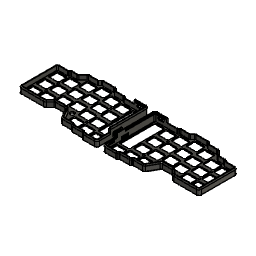
mriya-bumper-mjf-v1.01 (Autodesk Fusion 360 design; units mm, degrees)
Autodesk Fusion 360 part; units mm, degrees
(part 1 of 2)
sketch "mriya" plane through (0, 0, 0) normal (0, 0, 1) x (1, 0, 0)
  line L0 (-101.0213, 15.6719) -> (-94.7787, 21.9145) construction
  line L1 (-26.4858, 1.079) -> (-27.6142, 2.2074) construction
  line L2 (-138.1, 14.7932) -> (-103.1426, 14.7932) construction
  line L3 (-44.0716, 2.7932) -> (-29.0284, 2.7932) construction
  line L4 (-8.6, 0.4932) -> (-25.0716, 0.4932) construction
  line L5 (-64.4741, 6.1094) -> (-72.7517, 20.7608) construction
  line L6 (-45.4858, 3.379) -> (-46.6142, 4.5074) construction
  line L7 (-122.6142, 71.579) -> (-121.4858, 72.7074) construction
  line L8 (-101.0716, 81.2932) -> (-87.2284, 81.2932) construction
  line L9 (-138.1, 70.9932) -> (-124.0284, 70.9932) construction
  line L10 (-92.6574, 22.7932) -> (-76.2344, 22.7932) construction
  line L11 (-48.0284, 5.0932) -> (-62.7328, 5.0932) construction
  line L12 (-82.0716, 84.7932) -> (-64.7284, 84.7932) construction
  line L13 (-58.5716, 80.2932) -> (-45.7284, 80.2932) construction
  line L14 (-24.1, 19.4932) -> (-7.1, 19.4932) construction
  line L15 (-25.6, 20.9932) -> (-25.6, 77.9932) construction
  line L16 (-83.4858, 84.2074) -> (-85.8142, 81.879) construction
  line L17 (-63.3142, 84.2074) -> (-59.9858, 80.879) construction
  line L18 (-139.6, 69.4932) -> (-139.6, 16.2932) construction
  line L19 (-43.1858, 78.579) -> (-44.3142, 79.7074) construction
  line L20 (-99.4, 40.3932) -> (-99.4, 27.9932) construction
  line L21 (-98.6, 41.1932) -> (-86.2, 41.1932) construction
  line L22 (-98.6, 27.1932) -> (-86.2, 27.1932) construction
  line L23 (-85.4, 40.3932) -> (-85.4, 27.9932) construction
  line L24 (-42.4, 56.0932) -> (-42.4, 43.6932) construction
  line L25 (-41.6, 56.8932) -> (-29.2, 56.8932) construction
  line L26 (-41.6, 42.8932) -> (-29.2, 42.8932) construction
  line L27 (-28.4, 56.0932) -> (-28.4, 43.6932) construction
  line L28 (-61.4, 58.3932) -> (-61.4, 45.9932) construction
  line L29 (-60.6, 59.1932) -> (-48.2, 59.1932) construction
  line L30 (-60.6, 45.1932) -> (-48.2, 45.1932) construction
  line L31 (-47.4, 58.3932) -> (-47.4, 45.9932) construction
  line L32 (-137.4, 68.0932) -> (-137.4, 55.6932) construction
  line L33 (-136.6, 68.8932) -> (-124.2, 68.8932) construction
  line L34 (-136.6, 54.8932) -> (-124.2, 54.8932) construction
  line L35 (-123.4, 68.0932) -> (-123.4, 55.6932) construction
  line L36 (-61.4, 39.3932) -> (-61.4, 26.9932) construction
  line L37 (-60.6, 40.1932) -> (-48.2, 40.1932) construction
  line L38 (-60.6, 26.1932) -> (-48.2, 26.1932) construction
  line L39 (-47.4, 39.3932) -> (-47.4, 26.9932) construction
  line L40 (-42.4, 18.0932) -> (-42.4, 5.6932) construction
  line L41 (-41.6, 18.8932) -> (-29.2, 18.8932) construction
  line L42 (-41.6, 4.8932) -> (-29.2, 4.8932) construction
  line L43 (-28.4, 18.0932) -> (-28.4, 5.6932) construction
  line L44 (-23.4, 15.7932) -> (-23.4, 3.3932) construction
  line L45 (-22.6, 16.5932) -> (-10.2, 16.5932) construction
  line L46 (-22.6, 2.5932) -> (-10.2, 2.5932) construction
  line L47 (-9.4, 15.7932) -> (-9.4, 3.3932) construction
  line L48 (-137.4, 49.0932) -> (-137.4, 36.6932) construction
  line L49 (-136.6, 49.8932) -> (-124.2, 49.8932) construction
  line L50 (-136.6, 35.8932) -> (-124.2, 35.8932) construction
  line L51 (-123.4, 49.0932) -> (-123.4, 36.6932) construction
  line L52 (-118.4, 51.3932) -> (-118.4, 38.9932) construction
  line L53 (-117.6, 52.1932) -> (-105.2, 52.1932) construction
  line L54 (-117.6, 38.1932) -> (-105.2, 38.1932) construction
  line L55 (-104.4, 51.3932) -> (-104.4, 38.9932) construction
  line L56 (-137.4, 30.0932) -> (-137.4, 17.6932) construction
  line L57 (-136.6, 30.8932) -> (-124.2, 30.8932) construction
  line L58 (-136.6, 16.8932) -> (-124.2, 16.8932) construction
  line L59 (-123.4, 30.0932) -> (-123.4, 17.6932) construction
  line L60 (-61.4, 20.3932) -> (-61.4, 7.9932) construction
  line L61 (-60.6, 21.1932) -> (-48.2, 21.1932) construction
  line L62 (-60.6, 7.1932) -> (-48.2, 7.1932) construction
  line L63 (-47.4, 20.3932) -> (-47.4, 7.9932) construction
  line L64 (-80.4, 43.8932) -> (-80.4, 31.4932) construction
  line L65 (-79.6, 44.6932) -> (-67.2, 44.6932) construction
  line L66 (-79.6, 30.6932) -> (-67.2, 30.6932) construction
  line L67 (-66.4, 43.8932) -> (-66.4, 31.4932) construction
  line L68 (-80.4, 81.8932) -> (-80.4, 69.4932) construction
  line L69 (-79.6, 82.6932) -> (-67.2, 82.6932) construction
  line L70 (-79.6, 68.6932) -> (-67.2, 68.6932) construction
  line L71 (-66.4, 81.8932) -> (-66.4, 69.4932) construction
  line L72 (-42.4, 37.0932) -> (-42.4, 24.6932) construction
  line L73 (-41.6, 37.8932) -> (-29.2, 37.8932) construction
  line L74 (-41.6, 23.8932) -> (-29.2, 23.8932) construction
  line L75 (-28.4, 37.0932) -> (-28.4, 24.6932) construction
  line L76 (-118.4, 32.3932) -> (-118.4, 19.9932) construction
  line L77 (-117.6, 33.1932) -> (-105.2, 33.1932) construction
  line L78 (-117.6, 19.1932) -> (-105.2, 19.1932) construction
  line L79 (-104.4, 32.3932) -> (-104.4, 19.9932) construction
  line L80 (-61.4, 77.3932) -> (-61.4, 64.9932) construction
  line L81 (-60.6, 78.1932) -> (-48.2, 78.1932) construction
  line L82 (-60.6, 64.1932) -> (-48.2, 64.1932) construction
  line L83 (-47.4, 77.3932) -> (-47.4, 64.9932) construction
  line L84 (-42.4, 75.0932) -> (-42.4, 62.6932) construction
  line L85 (-41.6, 75.8932) -> (-29.2, 75.8932) construction
  line L86 (-41.6, 61.8932) -> (-29.2, 61.8932) construction
  line L87 (-28.4, 75.0932) -> (-28.4, 62.6932) construction
  line L88 (-118.4, 70.3932) -> (-118.4, 57.9932) construction
  line L89 (-117.6, 71.1932) -> (-105.2, 71.1932) construction
  line L90 (-117.6, 57.1932) -> (-105.2, 57.1932) construction
  line L91 (-104.4, 70.3932) -> (-104.4, 57.9932) construction
  line L92 (-99.4, 59.3932) -> (-99.4, 46.9932) construction
  line L93 (-98.6, 60.1932) -> (-86.2, 60.1932) construction
  line L94 (-98.6, 46.1932) -> (-86.2, 46.1932) construction
  line L95 (-85.4, 59.3932) -> (-85.4, 46.9932) construction
  line L96 (-80.4, 62.8932) -> (-80.4, 50.4932) construction
  line L97 (-79.6, 63.6932) -> (-67.2, 63.6932) construction
  line L98 (-79.6, 49.6932) -> (-67.2, 49.6932) construction
  line L99 (-66.4, 62.8932) -> (-66.4, 50.4932) construction
  line L100 (-99.4, 78.3932) -> (-99.4, 65.9932) construction
  line L101 (-98.6, 79.1932) -> (-86.2, 79.1932) construction
  line L102 (-98.6, 65.1932) -> (-86.2, 65.1932) construction
  line L103 (-85.4, 78.3932) -> (-85.4, 65.9932) construction
  circle A0 centre (-120.9, 53.5432) radius 1.6
  circle A1 centre (-120.9, 34.5432) radius 1.6
  circle A2 centre (-68.5, 23.5932) radius 3.5
  circle A3 centre (-44.9, 22.5432) radius 1.6
  circle A4 centre (-44.9, 60.5432) radius 1.6
  arc A5 (-43.1858, 78.579) -> (-41.7716, 77.9932) centre (-41.7716, 79.9932) ccw construction
  arc A6 (-44.3142, 79.7074) -> (-45.7284, 80.2932) centre (-45.7285, 78.2931) ccw construction
  arc A7 (-59.9858, 80.879) -> (-58.5716, 80.2932) centre (-58.5716, 82.2931) ccw construction
  arc A8 (-63.3142, 84.2074) -> (-64.7284, 84.7932) centre (-64.7285, 82.7931) ccw construction
  arc A9 (-82.0716, 84.7932) -> (-83.4858, 84.2074) centre (-82.0716, 82.7933) ccw construction
  arc A10 (-87.2284, 81.2932) -> (-85.8142, 81.879) centre (-87.2284, 83.2932) ccw construction
  arc A11 (-101.0716, 81.2932) -> (-102.4858, 80.7074) centre (-101.0716, 79.2933) ccw construction
  arc A12 (-120.0716, 73.2932) -> (-121.4858, 72.7074) centre (-120.0716, 71.2933) ccw construction
  arc A13 (-124.0284, 70.9932) -> (-122.6142, 71.579) centre (-124.0284, 72.9932) ccw construction
  arc A14 (-138.1, 70.9932) -> (-139.6, 69.4932) centre (-138.1, 69.4932) ccw construction
  arc A15 (-139.6, 16.2932) -> (-138.1, 14.7932) centre (-138.1, 16.2932) ccw construction
  arc A16 (-103.1426, 14.7932) -> (-101.0213, 15.6719) centre (-103.1426, 17.7931) ccw construction
  arc A17 (-92.6574, 22.7932) -> (-94.7787, 21.9145) centre (-92.6573, 19.7931) ccw construction
  arc A18 (-72.7517, 20.7608) -> (-76.2344, 22.7932) centre (-76.2344, 18.793) ccw construction
  arc A19 (-64.4741, 6.1094) -> (-62.7328, 5.0932) centre (-62.7328, 7.0932) ccw construction
  arc A20 (-46.6142, 4.5074) -> (-48.0284, 5.0932) centre (-48.0284, 3.0933) ccw construction
  arc A21 (-45.4858, 3.379) -> (-44.0716, 2.7932) centre (-44.0715, 4.7933) ccw construction
  arc A22 (-27.6142, 2.2074) -> (-29.0284, 2.7932) centre (-29.0284, 0.7933) ccw construction
  arc A23 (-26.4858, 1.079) -> (-25.0716, 0.4932) centre (-25.0715, 2.4933) ccw construction
  arc A24 (-8.6, 0.4932) -> (-7.1, 1.9932) centre (-8.6, 1.9932) ccw construction
  arc A25 (-25.6, 20.9932) -> (-24.1, 19.4932) centre (-24.1, 20.9932) ccw construction
  line L104 (-7.1, 1.9932) -> (-7.1, 76.4932) construction
  line L105 (-41.7716, 77.9932) -> (-8.6, 77.9932) construction
  arc A26 (-7.1, 76.4932) -> (-8.6, 77.9932) centre (-8.6, 76.4932) ccw construction
  arc A27 (-136.6, 68.8932) -> (-137.4, 68.0932) centre (-136.6, 68.0932) ccw construction
  arc A28 (-123.4, 68.0932) -> (-124.2, 68.8932) centre (-124.2, 68.0932) ccw construction
  arc A29 (-124.2, 54.8932) -> (-123.4, 55.6932) centre (-124.2, 55.6932) ccw construction
  arc A30 (-137.4, 55.6932) -> (-136.6, 54.8932) centre (-136.6, 55.6932) ccw construction
  arc A31 (-136.6, 49.8932) -> (-137.4, 49.0932) centre (-136.6, 49.0932) ccw construction
  arc A32 (-123.4, 49.0932) -> (-124.2, 49.8932) centre (-124.2, 49.0932) ccw construction
  arc A33 (-124.2, 35.8932) -> (-123.4, 36.6932) centre (-124.2, 36.6932) ccw construction
  arc A34 (-137.4, 36.6932) -> (-136.6, 35.8932) centre (-136.6, 36.6932) ccw construction
  arc A35 (-136.6, 30.8932) -> (-137.4, 30.0932) centre (-136.6, 30.0932) ccw construction
  arc A36 (-123.4, 30.0932) -> (-124.2, 30.8932) centre (-124.2, 30.0932) ccw construction
  arc A37 (-124.2, 16.8932) -> (-123.4, 17.6932) centre (-124.2, 17.6932) ccw construction
  arc A38 (-137.4, 17.6932) -> (-136.6, 16.8932) centre (-136.6, 17.6932) ccw construction
  arc A39 (-118.4, 19.9932) -> (-117.6, 19.1932) centre (-117.6, 19.9932) ccw construction
  arc A40 (-105.2, 19.1932) -> (-104.4, 19.9932) centre (-105.2, 19.9932) ccw construction
  arc A41 (-104.4, 32.3932) -> (-105.2, 33.1932) centre (-105.2, 32.3932) ccw construction
  arc A42 (-117.6, 33.1932) -> (-118.4, 32.3932) centre (-117.6, 32.3932) ccw construction
  arc A43 (-105.2, 38.1932) -> (-104.4, 38.9932) centre (-105.2, 38.9932) ccw construction
  arc A44 (-118.4, 38.9932) -> (-117.6, 38.1932) centre (-117.6, 38.9932) ccw construction
  arc A45 (-117.6, 52.1932) -> (-118.4, 51.3932) centre (-117.6, 51.3932) ccw construction
  arc A46 (-104.4, 51.3932) -> (-105.2, 52.1932) centre (-105.2, 51.3932) ccw construction
  arc A47 (-118.4, 57.9932) -> (-117.6, 57.1932) centre (-117.6, 57.9932) ccw construction
  arc A48 (-105.2, 57.1932) -> (-104.4, 57.9932) centre (-105.2, 57.9932) ccw construction
  arc A49 (-104.4, 70.3932) -> (-105.2, 71.1932) centre (-105.2, 70.3932) ccw construction
  arc A50 (-117.6, 71.1932) -> (-118.4, 70.3932) centre (-117.6, 70.3932) ccw construction
  arc A51 (-98.6, 79.1932) -> (-99.4, 78.3932) centre (-98.6, 78.3932) ccw construction
  arc A52 (-85.4, 78.3932) -> (-86.2, 79.1932) centre (-86.2, 78.3932) ccw construction
  arc A53 (-86.2, 65.1932) -> (-85.4, 65.9932) centre (-86.2, 65.9932) ccw construction
  arc A54 (-99.4, 65.9932) -> (-98.6, 65.1932) centre (-98.6, 65.9932) ccw construction
  arc A55 (-98.6, 60.1932) -> (-99.4, 59.3932) centre (-98.6, 59.3932) ccw construction
  arc A56 (-85.4, 59.3932) -> (-86.2, 60.1932) centre (-86.2, 59.3932) ccw construction
  arc A57 (-86.2, 46.1932) -> (-85.4, 46.9932) centre (-86.2, 46.9932) ccw construction
  arc A58 (-99.4, 46.9932) -> (-98.6, 46.1932) centre (-98.6, 46.9932) ccw construction
  arc A59 (-98.6, 41.1932) -> (-99.4, 40.3932) centre (-98.6, 40.3932) ccw construction
  arc A60 (-99.4, 27.9932) -> (-98.6, 27.1932) centre (-98.6, 27.9932) ccw construction
  arc A61 (-86.2, 27.1932) -> (-85.4, 27.9932) centre (-86.2, 27.9932) ccw construction
  arc A62 (-85.4, 40.3932) -> (-86.2, 41.1932) centre (-86.2, 40.3932) ccw construction
  arc A63 (-80.4, 31.4932) -> (-79.6, 30.6932) centre (-79.6, 31.4932) ccw construction
  arc A64 (-79.6, 44.6932) -> (-80.4, 43.8932) centre (-79.6, 43.8932) ccw construction
  arc A65 (-66.4, 43.8932) -> (-67.2, 44.6932) centre (-67.2, 43.8932) ccw construction
  arc A66 (-67.2, 30.6932) -> (-66.4, 31.4932) centre (-67.2, 31.4932) ccw construction
  arc A67 (-67.2, 49.6932) -> (-66.4, 50.4932) centre (-67.2, 50.4932) ccw construction
  arc A68 (-80.4, 50.4932) -> (-79.6, 49.6932) centre (-79.6, 50.4932) ccw construction
  arc A69 (-79.6, 63.6932) -> (-80.4, 62.8932) centre (-79.6, 62.8932) ccw construction
  arc A70 (-66.4, 62.8932) -> (-67.2, 63.6932) centre (-67.2, 62.8932) ccw construction
  arc A71 (-67.2, 68.6932) -> (-66.4, 69.4932) centre (-67.2, 69.4932) ccw construction
  arc A72 (-80.4, 69.4932) -> (-79.6, 68.6932) centre (-79.6, 69.4932) ccw construction
  arc A73 (-79.6, 82.6932) -> (-80.4, 81.8932) centre (-79.6, 81.8932) ccw construction
  arc A74 (-66.4, 81.8932) -> (-67.2, 82.6932) centre (-67.2, 81.8932) ccw construction
  arc A75 (-60.6, 78.1932) -> (-61.4, 77.3932) centre (-60.6, 77.3932) ccw construction
  arc A76 (-61.4, 64.9932) -> (-60.6, 64.1932) centre (-60.6, 64.9932) ccw construction
  arc A77 (-48.2, 64.1932) -> (-47.4, 64.9932) centre (-48.2, 64.9932) ccw construction
  arc A78 (-47.4, 77.3932) -> (-48.2, 78.1932) centre (-48.2, 77.3932) ccw construction
  arc A79 (-47.4, 58.3932) -> (-48.2, 59.1932) centre (-48.2, 58.3932) ccw construction
  arc A80 (-60.6, 59.1932) -> (-61.4, 58.3932) centre (-60.6, 58.3932) ccw construction
  arc A81 (-61.4, 45.9932) -> (-60.6, 45.1932) centre (-60.6, 45.9932) ccw construction
  arc A82 (-48.2, 45.1932) -> (-47.4, 45.9932) centre (-48.2, 45.9932) ccw construction
  arc A83 (-47.4, 39.3932) -> (-48.2, 40.1932) centre (-48.2, 39.3932) ccw construction
  arc A84 (-60.6, 40.1932) -> (-61.4, 39.3932) centre (-60.6, 39.3932) ccw construction
  arc A85 (-61.4, 26.9932) -> (-60.6, 26.1932) centre (-60.6, 26.9932) ccw construction
  arc A86 (-48.2, 26.1932) -> (-47.4, 26.9932) centre (-48.2, 26.9932) ccw construction
  arc A87 (-47.4, 20.3932) -> (-48.2, 21.1932) centre (-48.2, 20.3932) ccw construction
  arc A88 (-60.6, 21.1932) -> (-61.4, 20.3932) centre (-60.6, 20.3932) ccw construction
  arc A89 (-61.4, 7.9932) -> (-60.6, 7.1932) centre (-60.6, 7.9932) ccw construction
  arc A90 (-48.2, 7.1932) -> (-47.4, 7.9932) centre (-48.2, 7.9932) ccw construction
  arc A91 (-42.4, 5.6932) -> (-41.6, 4.8932) centre (-41.6, 5.6932) ccw construction
  arc A92 (-29.2, 4.8932) -> (-28.4, 5.6932) centre (-29.2, 5.6932) ccw construction
  arc A93 (-28.4, 18.0932) -> (-29.2, 18.8932) centre (-29.2, 18.0932) ccw construction
  arc A94 (-41.6, 18.8932) -> (-42.4, 18.0932) centre (-41.6, 18.0932) ccw construction
  arc A95 (-23.4, 3.3932) -> (-22.6, 2.5932) centre (-22.6, 3.3932) ccw construction
  arc A96 (-10.2, 2.5932) -> (-9.4, 3.3932) centre (-10.2, 3.3932) ccw construction
  arc A97 (-9.4, 15.7932) -> (-10.2, 16.5932) centre (-10.2, 15.7932) ccw construction
  arc A98 (-22.6, 16.5932) -> (-23.4, 15.7932) centre (-22.6, 15.7932) ccw construction
  arc A99 (-29.2, 23.8932) -> (-28.4, 24.6932) centre (-29.2, 24.6932) ccw construction
  arc A100 (-42.4, 24.6932) -> (-41.6, 23.8932) centre (-41.6, 24.6932) ccw construction
  arc A101 (-41.6, 37.8932) -> (-42.4, 37.0932) centre (-41.6, 37.0932) ccw construction
  arc A102 (-28.4, 37.0932) -> (-29.2, 37.8932) centre (-29.2, 37.0932) ccw construction
  arc A103 (-29.2, 42.8932) -> (-28.4, 43.6932) centre (-29.2, 43.6932) ccw construction
  arc A104 (-42.4, 43.6932) -> (-41.6, 42.8932) centre (-41.6, 43.6932) ccw construction
  arc A105 (-41.6, 56.8932) -> (-42.4, 56.0932) centre (-41.6, 56.0932) ccw construction
  arc A106 (-28.4, 56.0932) -> (-29.2, 56.8932) centre (-29.2, 56.0932) ccw construction
  arc A107 (-29.2, 61.8932) -> (-28.4, 62.6932) centre (-29.2, 62.6932) ccw construction
  arc A108 (-42.4, 62.6932) -> (-41.6, 61.8932) centre (-41.6, 62.6932) ccw construction
  arc A109 (-41.6, 75.8932) -> (-42.4, 75.0932) centre (-41.6, 75.0932) ccw construction
  arc A110 (-28.4, 75.0932) -> (-29.2, 75.8932) centre (-29.2, 75.0932) ccw construction
  line L106 (-122.6496, 71.6144) -> (-121.5212, 72.7428)
  arc A111 (-120.0716, 73.3432) -> (-121.5212, 72.7428) centre (-120.0716, 71.2933) ccw
  arc A112 (-101.0716, 81.3432) -> (-102.5212, 80.7428) centre (-101.0716, 79.2933) ccw
  line L107 (-101.0716, 81.3432) -> (-87.2284, 81.3432)
  arc A113 (-87.2284, 81.3432) -> (-85.8496, 81.9144) centre (-87.2284, 83.2932) ccw
  line L108 (-83.5212, 84.2428) -> (-85.8496, 81.9144)
  arc A114 (-82.0716, 84.8432) -> (-83.5212, 84.2428) centre (-82.0716, 82.7933) ccw
  line L109 (-82.0716, 84.8432) -> (-64.7284, 84.8432)
  arc A115 (-63.2788, 84.2427) -> (-64.7284, 84.8432) centre (-64.7285, 82.7931) ccw
  line L110 (-63.2788, 84.2427) -> (-59.9504, 80.9144)
  arc A116 (-59.9504, 80.9144) -> (-58.5716, 80.3432) centre (-58.5716, 82.2931) ccw
  line L111 (-58.5716, 80.3432) -> (-45.7284, 80.3432)
  arc A117 (-44.2788, 79.7427) -> (-45.7284, 80.3432) centre (-45.7285, 78.2931) ccw
  line L112 (-43.1504, 78.6144) -> (-44.2788, 79.7427)
  arc A118 (-43.1504, 78.6144) -> (-41.7716, 78.0432) centre (-41.7716, 79.9932) ccw
  line L113 (-41.7716, 78.0432) -> (-8.6, 78.0432)
  arc A119 (-7.05, 76.4932) -> (-8.6, 78.0432) centre (-8.6, 76.4932) ccw
  line L114 (-7.05, 1.9932) -> (-7.05, 76.4932)
  arc A120 (-8.6, 0.4432) -> (-7.05, 1.9932) centre (-8.6, 1.9932) ccw
  line L115 (-8.6, 0.4432) -> (-25.0716, 0.4432)
  arc A121 (-26.5212, 1.0437) -> (-25.0716, 0.4432) centre (-25.0715, 2.4933) ccw
  line L116 (-26.5212, 1.0437) -> (-27.6496, 2.172)
  arc A122 (-27.6496, 2.172) -> (-29.0284, 2.7432) centre (-29.0284, 0.7933) ccw
  line L117 (-44.0716, 2.7432) -> (-29.0284, 2.7432)
  arc A123 (-45.5212, 3.3437) -> (-44.0716, 2.7432) centre (-44.0715, 4.7933) ccw
  line L118 (-45.5212, 3.3437) -> (-46.6496, 4.472)
  arc A124 (-46.6496, 4.472) -> (-48.0284, 5.0432) centre (-48.0284, 3.0933) ccw
  line L119 (-48.0284, 5.0432) -> (-62.7328, 5.0432)
  arc A125 (-64.5176, 6.0848) -> (-62.7328, 5.0432) centre (-62.7328, 7.0932) ccw
  line L120 (-64.5176, 6.0848) -> (-72.7952, 20.7362)
  arc A126 (-72.7952, 20.7362) -> (-76.2344, 22.7432) centre (-76.2344, 18.793) ccw
  line L121 (-92.6574, 22.7432) -> (-76.2344, 22.7432)
  arc A127 (-92.6574, 22.7432) -> (-94.7433, 21.8791) centre (-92.6573, 19.7931) ccw
  line L122 (-100.9859, 15.6365) -> (-94.7433, 21.8791)
  arc A128 (-103.1426, 14.7432) -> (-100.9859, 15.6365) centre (-103.1426, 17.7931) ccw
  line L123 (-138.1, 14.7432) -> (-103.1426, 14.7432)
  arc A129 (-139.65, 16.2932) -> (-138.1, 14.7432) centre (-138.1, 16.2932) ccw
  line L124 (-139.65, 69.4932) -> (-139.65, 16.2932)
  arc A130 (-138.1, 71.0432) -> (-139.65, 69.4932) centre (-138.1, 69.4932) ccw
  line L125 (-138.1, 71.0432) -> (-124.0284, 71.0432)
  arc A131 (-124.0284, 71.0432) -> (-122.6496, 71.6144) centre (-124.0284, 72.9932) ccw
  line L126 (-82.7136, 87.3432) -> (-64.0864, 87.3432)
  arc A132 (-4.55, 76.4932) -> (-8.6, 80.5432) centre (-8.6, 76.4932) ccw
  line L127 (-4.55, 1.9932) -> (-4.55, 76.4932)
  arc A133 (-8.6, -2.0568) -> (-4.55, 1.9932) centre (-8.6, 1.9932) ccw
  line L128 (-8.6, -2.0568) -> (-25.7136, -2.0568)
  line L129 (-138.1, 12.2432) -> (-102.7077, 12.2432)
  arc A134 (-142.15, 16.2932) -> (-138.1, 12.2432) centre (-138.1, 16.2932) ccw
  line L130 (-142.15, 69.4932) -> (-142.15, 16.2932)
  arc A135 (-138.1, 73.5432) -> (-142.15, 69.4932) centre (-138.1, 69.4932) ccw
  circle A136 centre (-22.6, 22.4932) radius 1.1 construction
  circle A137 centre (-10.1, 22.4932) radius 1.1 construction
  line L131 (-7.05, 19.2932) -> (-4.55, 19.2932)
  line L132 (-25.8, 78.0432) -> (-25.8, 80.5432)
  line L133 (-23.1, 77.8432) -> (-23.1, 78.0432)
  line L134 (-22.5, 77.2432) -> (-8.65, 77.2432)
  line L135 (-7.25, 31.4932) -> (-7.05, 31.4932)
  line L136 (-7.85, 32.0932) -> (-7.85, 76.4432)
  arc A138 (-7.85, 76.4432) -> (-8.65, 77.2432) centre (-8.65, 76.4432) ccw
  arc A139 (-23.1, 77.8432) -> (-22.5, 77.2432) centre (-22.5, 77.8432) ccw
  arc A140 (-7.85, 32.0932) -> (-7.25, 31.4932) centre (-7.25, 32.0932) ccw
  line L137 (-7.05, 14.5932) -> (-7.25, 14.5932)
  line L138 (-7.85, 13.9932) -> (-7.85, 5.1932)
  line L139 (-7.25, 4.5932) -> (-7.05, 4.5932)
  arc A141 (-7.25, 14.5932) -> (-7.85, 13.9932) centre (-7.25, 13.9932) ccw
  arc A142 (-7.85, 5.1932) -> (-7.25, 4.5932) centre (-7.25, 5.1932) ccw
  line L140 (-102.4858, 80.7074) -> (-109.0213, 74.1719) construction
  line L141 (-120.0716, 73.2932) -> (-111.1426, 73.2932) construction
  line L142 (-102.5212, 80.7428) -> (-109.0567, 74.2072)
  line L143 (-111.1426, 73.3432) -> (-120.0716, 73.3432)
  arc A143 (-111.1426, 73.3432) -> (-109.0567, 74.2072) centre (-111.1426, 76.2932) ccw
  arc A144 (-111.1426, 73.2932) -> (-109.0213, 74.1719) centre (-111.1426, 76.2932) ccw construction
  line L144 (-92.0153, 20.2432) -> (-77.1389, 20.2432)
  arc A145 (-92.0153, 20.2432) -> (-93.4295, 19.6574) centre (-92.0153, 18.2432) ccw
  arc A146 (-74.5269, 18.7189) -> (-77.1389, 20.2432) centre (-77.1389, 17.2432) ccw
  line L145 (-111.3705, 75.8432) -> (-120.7136, 75.8432)
  line L146 (-138.1, 73.5432) -> (-124.6705, 73.5432)
  line L147 (-101.7136, 83.8432) -> (-87.8705, 83.8432)
  line L148 (-57.9295, 82.8432) -> (-45.0864, 82.8432)
  line L149 (-41.1295, 80.5432) -> (-8.6, 80.5432)
  line L150 (-44.7136, 0.2432) -> (-29.6705, 0.2432)
  line L151 (-63.3456, 2.5432) -> (-48.6705, 2.5432)
  arc A147 (-64.7284, 82.7932) -> (-64.7285, 82.7932) centre (-64.7285, 82.7931) ccw
  arc A148 (-45.7284, 78.2932) -> (-45.7285, 78.2932) centre (-45.7285, 78.2931) ccw
  arc A149 (-25.0716, 2.4932) -> (-25.0715, 2.4932) centre (-25.0715, 2.4933) ccw
  arc A150 (-44.0716, 4.7932) -> (-44.0715, 4.7932) centre (-44.0715, 4.7933) ccw
  line L152 (-138.9, 56.8932) -> (-138.9, 66.8932)
  line L153 (-136.9, 68.8932) -> (-123.9, 68.8932)
  arc A151 (-121.9, 66.8932) -> (-123.9, 68.8932) centre (-123.9, 66.8932) ccw
  arc A152 (-138.9, 56.8932) -> (-136.9, 54.8932) centre (-136.9, 56.8932) ccw
  arc A153 (-136.9, 68.8932) -> (-138.9, 66.8932) centre (-136.9, 66.8932) ccw
  arc A154 (-138.9, 37.8932) -> (-136.9, 35.8932) centre (-136.9, 37.8932) ccw
  line L154 (-138.9, 37.8932) -> (-138.9, 47.8932)
  arc A155 (-136.9, 49.8932) -> (-138.9, 47.8932) centre (-136.9, 47.8932) ccw
  line L155 (-136.9, 49.8932) -> (-123.9, 49.8932)
  arc A156 (-121.9, 47.8932) -> (-123.9, 49.8932) centre (-123.9, 47.8932) ccw
  arc A157 (-123.9, 16.8932) -> (-121.9, 18.8932) centre (-123.9, 18.8932) ccw
  line L156 (-123.9, 16.8932) -> (-136.9, 16.8932)
  arc A158 (-138.9, 18.8932) -> (-136.9, 16.8932) centre (-136.9, 18.8932) ccw
  line L157 (-138.9, 18.8932) -> (-138.9, 28.8932)
  arc A159 (-136.9, 30.8932) -> (-138.9, 28.8932) centre (-136.9, 28.8932) ccw
  line L158 (-136.9, 30.8932) -> (-123.9, 30.8932)
  arc A160 (-121.9, 28.8932) -> (-123.9, 30.8932) centre (-123.9, 28.8932) ccw
  line L159 (-121.9, 28.8932) -> (-121.9, 18.8932)
  arc A161 (-104.9, 57.1932) -> (-102.9, 59.1932) centre (-104.9, 59.1932) ccw
  line L160 (-104.9, 57.1932) -> (-117.9, 57.1932)
  arc A162 (-119.9, 59.1932) -> (-117.9, 57.1932) centre (-117.9, 59.1932) ccw
  line L161 (-119.9, 59.1932) -> (-119.9, 69.1932)
  arc A163 (-117.9, 71.1932) -> (-119.9, 69.1932) centre (-117.9, 69.1932) ccw
  line L162 (-117.9, 71.1932) -> (-104.9, 71.1932)
  arc A164 (-102.9, 69.1932) -> (-104.9, 71.1932) centre (-104.9, 69.1932) ccw
  line L163 (-102.9, 69.1932) -> (-102.9, 59.1932)
  arc A165 (-104.9, 38.1932) -> (-102.9, 40.1932) centre (-104.9, 40.1932) ccw
  line L164 (-104.9, 38.1932) -> (-117.9, 38.1932)
  arc A166 (-119.9, 40.1932) -> (-117.9, 38.1932) centre (-117.9, 40.1932) ccw
  arc A167 (-102.9, 50.1932) -> (-104.9, 52.1932) centre (-104.9, 50.1932) ccw
  line L165 (-102.9, 50.1932) -> (-102.9, 40.1932)
  arc A168 (-104.9, 19.1932) -> (-102.9, 21.1932) centre (-104.9, 21.1932) ccw
  line L166 (-104.9, 19.1932) -> (-117.9, 19.1932)
  arc A169 (-119.9, 21.1932) -> (-117.9, 19.1932) centre (-117.9, 21.1932) ccw
  arc A170 (-102.9, 31.1932) -> (-104.9, 33.1932) centre (-104.9, 31.1932) ccw
  line L167 (-102.9, 31.1932) -> (-102.9, 21.1932)
  arc A171 (-85.9, 65.1932) -> (-83.9, 67.1932) centre (-85.9, 67.1932) ccw
  line L168 (-85.9, 65.1932) -> (-98.9, 65.1932)
  arc A172 (-100.9, 67.1932) -> (-98.9, 65.1932) centre (-98.9, 67.1932) ccw
  line L169 (-100.9, 67.1932) -> (-100.9, 77.1932)
  arc A173 (-98.9, 79.1932) -> (-100.9, 77.1932) centre (-98.9, 77.1932) ccw
  line L170 (-98.9, 79.1932) -> (-85.9, 79.1932)
  arc A174 (-83.9, 77.1932) -> (-85.9, 79.1932) centre (-85.9, 77.1932) ccw
  line L171 (-83.9, 77.1932) -> (-83.9, 67.1932)
  arc A175 (-85.9, 46.1932) -> (-83.9, 48.1932) centre (-85.9, 48.1932) ccw
  line L172 (-85.9, 46.1932) -> (-98.9, 46.1932)
  arc A176 (-100.9, 48.1932) -> (-98.9, 46.1932) centre (-98.9, 48.1932) ccw
  line L173 (-100.9, 48.1932) -> (-100.9, 58.1932)
  arc A177 (-98.9, 60.1932) -> (-100.9, 58.1932) centre (-98.9, 58.1932) ccw
  line L174 (-98.9, 60.1932) -> (-85.9, 60.1932)
  arc A178 (-83.9, 58.1932) -> (-85.9, 60.1932) centre (-85.9, 58.1932) ccw
  line L175 (-83.9, 58.1932) -> (-83.9, 48.1932)
  arc A179 (-85.9, 27.1932) -> (-83.9, 29.1932) centre (-85.9, 29.1932) ccw
  line L176 (-85.9, 27.1932) -> (-98.9, 27.1932)
  arc A180 (-100.9, 29.1932) -> (-98.9, 27.1932) centre (-98.9, 29.1932) ccw
  line L177 (-100.9, 29.1932) -> (-100.9, 39.1932)
  arc A181 (-98.9, 41.1932) -> (-100.9, 39.1932) centre (-98.9, 39.1932) ccw
  line L178 (-98.9, 41.1932) -> (-85.9, 41.1932)
  arc A182 (-83.9, 39.1932) -> (-85.9, 41.1932) centre (-85.9, 39.1932) ccw
  line L179 (-83.9, 39.1932) -> (-83.9, 29.1932)
  arc A183 (-66.9, 30.6932) -> (-64.9, 32.6932) centre (-66.9, 32.6932) ccw
  line L180 (-66.9, 30.6932) -> (-79.9, 30.6932)
  arc A184 (-81.9, 32.6932) -> (-79.9, 30.6932) centre (-79.9, 32.6932) ccw
  line L181 (-81.9, 32.6932) -> (-81.9, 42.6932)
  arc A185 (-79.9, 44.6932) -> (-81.9, 42.6932) centre (-79.9, 42.6932) ccw
  line L182 (-79.9, 44.6932) -> (-66.9, 44.6932)
  arc A186 (-64.9, 42.6932) -> (-66.9, 44.6932) centre (-66.9, 42.6932) ccw
  line L183 (-64.9, 42.6932) -> (-64.9, 32.6932)
  arc A187 (-66.9, 49.6932) -> (-64.9, 51.6932) centre (-66.9, 51.6932) ccw
  line L184 (-66.9, 49.6932) -> (-79.9, 49.6932)
  arc A188 (-81.9, 51.6932) -> (-79.9, 49.6932) centre (-79.9, 51.6932) ccw
  line L185 (-81.9, 51.6932) -> (-81.9, 61.6932)
  arc A189 (-79.9, 63.6932) -> (-81.9, 61.6932) centre (-79.9, 61.6932) ccw
  line L186 (-79.9, 63.6932) -> (-66.9, 63.6932)
  arc A190 (-64.9, 61.6932) -> (-66.9, 63.6932) centre (-66.9, 61.6932) ccw
  line L187 (-64.9, 61.6932) -> (-64.9, 51.6932)
  arc A191 (-66.9, 68.6932) -> (-64.9, 70.6932) centre (-66.9, 70.6932) ccw
  line L188 (-66.9, 68.6932) -> (-79.9, 68.6932)
  arc A192 (-81.9, 70.6932) -> (-79.9, 68.6932) centre (-79.9, 70.6932) ccw
  line L189 (-81.9, 70.6932) -> (-81.9, 80.6932)
  arc A193 (-79.9, 82.6932) -> (-81.9, 80.6932) centre (-79.9, 80.6932) ccw
  line L190 (-79.9, 82.6932) -> (-66.9, 82.6932)
  arc A194 (-64.9, 80.6932) -> (-66.9, 82.6932) centre (-66.9, 80.6932) ccw
  line L191 (-64.9, 80.6932) -> (-64.9, 70.6932)
  arc A195 (-47.9, 26.1932) -> (-45.9, 28.1932) centre (-47.9, 28.1932) ccw
  line L192 (-47.9, 26.1932) -> (-60.9, 26.1932)
  arc A196 (-62.9, 28.1932) -> (-60.9, 26.1932) centre (-60.9, 28.1932) ccw
  line L193 (-62.9, 28.1932) -> (-62.9, 38.1932)
  arc A197 (-60.9, 40.1932) -> (-62.9, 38.1932) centre (-60.9, 38.1932) ccw
  line L194 (-60.9, 40.1932) -> (-47.9, 40.1932)
  arc A198 (-45.9, 38.1932) -> (-47.9, 40.1932) centre (-47.9, 38.1932) ccw
  line L195 (-45.9, 38.1932) -> (-45.9, 28.1932)
  arc A199 (-47.9, 45.1932) -> (-45.9, 47.1932) centre (-47.9, 47.1932) ccw
  line L196 (-47.9, 45.1932) -> (-60.9, 45.1932)
  arc A200 (-62.9, 47.1932) -> (-60.9, 45.1932) centre (-60.9, 47.1932) ccw
  line L197 (-62.9, 47.1932) -> (-62.9, 57.1932)
  arc A201 (-60.9, 59.1932) -> (-62.9, 57.1932) centre (-60.9, 57.1932) ccw
  arc A202 (-47.9, 64.1932) -> (-45.9, 66.1932) centre (-47.9, 66.1932) ccw
  line L198 (-47.9, 64.1932) -> (-60.9, 64.1932)
  arc A203 (-62.9, 66.1932) -> (-60.9, 64.1932) centre (-60.9, 66.1932) ccw
  line L199 (-62.9, 66.1932) -> (-62.9, 76.1932)
  arc A204 (-60.9, 78.1932) -> (-62.9, 76.1932) centre (-60.9, 76.1932) ccw
  line L200 (-60.9, 78.1932) -> (-47.9, 78.1932)
  arc A205 (-45.9, 76.1932) -> (-47.9, 78.1932) centre (-47.9, 76.1932) ccw
  line L201 (-45.9, 76.1932) -> (-45.9, 66.1932)
  arc A206 (-47.9, 7.1932) -> (-45.9, 9.1932) centre (-47.9, 9.1932) ccw
  line L202 (-47.9, 7.1932) -> (-60.9, 7.1932)
  arc A207 (-62.9, 9.1932) -> (-60.9, 7.1932) centre (-60.9, 9.1932) ccw
  line L203 (-62.9, 9.1932) -> (-62.9, 19.1932)
  arc A208 (-60.9, 21.1932) -> (-62.9, 19.1932) centre (-60.9, 19.1932) ccw
  arc A209 (-28.9, 4.8932) -> (-26.9, 6.8932) centre (-28.9, 6.8932) ccw
  line L204 (-28.9, 4.8932) -> (-41.9, 4.8932)
  arc A210 (-43.9, 6.8932) -> (-41.9, 4.8932) centre (-41.9, 6.8932) ccw
  line L205 (-43.9, 6.8932) -> (-43.9, 16.8932)
  arc A211 (-41.9, 18.8932) -> (-43.9, 16.8932) centre (-41.9, 16.8932) ccw
  line L206 (-41.9, 18.8932) -> (-28.9, 18.8932)
  arc A212 (-26.9, 16.8932) -> (-28.9, 18.8932) centre (-28.9, 16.8932) ccw
  line L207 (-26.9, 16.8932) -> (-26.9, 6.8932)
  arc A213 (-28.9, 23.8932) -> (-26.9, 25.8932) centre (-28.9, 25.8932) ccw
  arc A214 (-41.9, 37.8932) -> (-43.9, 35.8932) centre (-41.9, 35.8932) ccw
  line L208 (-41.9, 37.8932) -> (-28.9, 37.8932)
  arc A215 (-26.9, 35.8932) -> (-28.9, 37.8932) centre (-28.9, 35.8932) ccw
  line L209 (-26.9, 35.8932) -> (-26.9, 25.8932)
  arc A216 (-28.9, 42.8932) -> (-26.9, 44.8932) centre (-28.9, 44.8932) ccw
  line L210 (-28.9, 42.8932) -> (-41.9, 42.8932)
  arc A217 (-43.9, 44.8932) -> (-41.9, 42.8932) centre (-41.9, 44.8932) ccw
  line L211 (-43.9, 44.8932) -> (-43.9, 54.8932)
  arc A218 (-41.9, 56.8932) -> (-43.9, 54.8932) centre (-41.9, 54.8932) ccw
  line L212 (-41.9, 56.8932) -> (-28.9, 56.8932)
  arc A219 (-26.9, 54.8932) -> (-28.9, 56.8932) centre (-28.9, 54.8932) ccw
  line L213 (-26.9, 54.8932) -> (-26.9, 44.8932)
  arc A220 (-28.9, 61.8932) -> (-26.9, 63.8932) centre (-28.9, 63.8932) ccw
  line L214 (-43.9, 64.3145) -> (-43.9, 73.8932)
  arc A221 (-41.9, 75.8932) -> (-43.9, 73.8932) centre (-41.9, 73.8932) ccw
  line L215 (-41.9, 75.8932) -> (-28.9, 75.8932)
  arc A222 (-26.9, 73.8932) -> (-28.9, 75.8932) centre (-28.9, 73.8932) ccw
  line L216 (-26.9, 73.8932) -> (-26.9, 63.8932)
  arc A223 (-9.9, 2.5932) -> (-7.9, 4.5932) centre (-9.9, 4.5932) ccw
  line L217 (-9.9, 2.5932) -> (-22.9, 2.5932)
  arc A224 (-24.9, 4.5932) -> (-22.9, 2.5932) centre (-22.9, 4.5932) ccw
  line L218 (-24.9, 4.5932) -> (-24.9, 14.5932)
  arc A225 (-22.9, 16.5932) -> (-24.9, 14.5932) centre (-22.9, 14.5932) ccw
  line L219 (-22.9, 16.5932) -> (-9.9, 16.5932)
  arc A226 (-7.9, 14.5932) -> (-9.9, 16.5932) centre (-9.9, 14.5932) ccw
  line L220 (-7.9, 14.5932) -> (-7.9, 4.5932)
  arc A227 (-9.9, 19.8932) -> (-7.9, 21.8932) centre (-9.9, 21.8932) ccw
  line L221 (-9.9, 19.8932) -> (-22.9, 19.8932)
  arc A228 (-24.9, 21.8932) -> (-22.9, 19.8932) centre (-22.9, 21.8932) ccw
  line L222 (-24.9, 21.8932) -> (-24.9, 73.8932)
  arc A229 (-22.9, 75.8932) -> (-24.9, 73.8932) centre (-22.9, 73.8932) ccw
  line L223 (-22.9, 75.8932) -> (-9.9, 75.8932)
  arc A230 (-7.9, 73.8932) -> (-9.9, 75.8932) centre (-9.9, 73.8932) ccw
  line L224 (-7.9, 73.8932) -> (-7.9, 21.8932)
  arc A231 (-120.7136, 75.8432) -> (-122.8349, 74.9645) centre (-120.7136, 72.8432) ccw
  line L225 (-123.9634, 73.8361) -> (-122.8349, 74.9645)
  arc A232 (-124.6705, 73.5432) -> (-123.9634, 73.8361) centre (-124.6705, 74.5432) ccw
  line L226 (-110.6634, 76.1361) -> (-103.8349, 82.9645)
  arc A233 (-111.3705, 75.8432) -> (-110.6634, 76.1361) centre (-111.3705, 76.8432) ccw
  arc A234 (-101.7136, 83.8432) -> (-103.8349, 82.9645) centre (-101.7136, 80.8432) ccw
  line L227 (-87.1634, 84.1361) -> (-84.8349, 86.4645)
  arc A235 (-87.8705, 83.8432) -> (-87.1634, 84.1361) centre (-87.8705, 84.8432) ccw
  arc A236 (-82.7136, 87.3432) -> (-84.8349, 86.4645) centre (-82.7136, 84.3432) ccw
  line L228 (-58.6367, 83.1361) -> (-61.9651, 86.4645)
  arc A237 (-61.9651, 86.4645) -> (-64.0864, 87.3432) centre (-64.0864, 84.3432) ccw
  arc A238 (-58.6367, 83.1361) -> (-57.9295, 82.8432) centre (-57.9295, 83.8432) ccw
  line L229 (-41.8367, 80.8361) -> (-42.9651, 81.9645)
  arc A239 (-42.9651, 81.9645) -> (-45.0864, 82.8432) centre (-45.0864, 79.8432) ccw
  arc A240 (-41.8367, 80.8361) -> (-41.1295, 80.5432) centre (-41.1295, 81.5432) ccw
  line L230 (-47.9633, 2.2503) -> (-46.8349, 1.1219)
  arc A241 (-47.9633, 2.2503) -> (-48.6705, 2.5432) centre (-48.6705, 1.5432) ccw
  arc A242 (-46.8349, 1.1219) -> (-44.7136, 0.2432) centre (-44.7136, 3.2432) ccw
  line L231 (-74.5269, 18.7189) -> (-66.3929, 4.3216)
  arc A243 (-66.3929, 4.3216) -> (-63.3456, 2.5432) centre (-63.3456, 6.0432) ccw
  line L232 (-99.5257, 13.5612) -> (-93.4295, 19.6574)
  arc A244 (-102.7077, 12.2432) -> (-99.5257, 13.5612) centre (-102.7077, 16.7432) ccw
  line L233 (-28.9633, -0.0497) -> (-27.8349, -1.1781)
  arc A245 (-28.9633, -0.0497) -> (-29.6705, 0.2432) centre (-29.6705, -0.7568) ccw
  arc A246 (-27.8349, -1.1781) -> (-25.7136, -2.0568) centre (-25.7136, 0.9432) ccw
  line L234 (-43.9, 26.3145) -> (-43.9, 35.8932)
  line L235 (-28.9, 23.8932) -> (-41.4787, 23.8932)
  line L236 (-43.4607, 25.2539) -> (-42.5393, 24.3325)
  line L237 (-60.9, 21.1932) -> (-48.3213, 21.1932)
  line L238 (-45.9, 18.7719) -> (-45.9, 9.1932)
  line L239 (-47.2607, 20.7539) -> (-46.3393, 19.8325)
  line L240 (-60.9, 59.1932) -> (-48.3213, 59.1932)
  line L241 (-45.9, 56.7719) -> (-45.9, 47.1932)
  line L242 (-28.9, 61.8932) -> (-41.4787, 61.8932)
  line L243 (-47.2607, 58.7539) -> (-46.3393, 57.8325)
  line L244 (-42.5393, 62.3325) -> (-43.4607, 63.2539)
  line L245 (-121.9, 66.8932) -> (-121.9, 57.3145)
  line L246 (-124.3213, 54.8932) -> (-136.9, 54.8932)
  line L247 (-117.4787, 52.1932) -> (-104.9, 52.1932)
  line L248 (-119.9, 40.1932) -> (-119.9, 49.7719)
  line L249 (-123.2607, 55.3325) -> (-122.3393, 56.2539)
  line L250 (-118.5393, 51.7539) -> (-119.4607, 50.8325)
  line L251 (-119.9, 21.1932) -> (-119.9, 30.7719)
  line L252 (-117.4787, 33.1932) -> (-104.9, 33.1932)
  line L253 (-121.9, 47.8932) -> (-121.9, 38.3145)
  line L254 (-124.3213, 35.8932) -> (-136.9, 35.8932)
  line L255 (-123.2607, 36.3325) -> (-122.3393, 37.2539)
  line L256 (-119.4607, 31.8325) -> (-118.5393, 32.7539)
  arc A247 (-43.9, 26.3145) -> (-43.4607, 25.2539) centre (-42.4, 26.3145) ccw
  arc A248 (-42.5393, 24.3325) -> (-41.4787, 23.8932) centre (-41.4787, 25.3932) ccw
  arc A249 (-47.2607, 20.7539) -> (-48.3213, 21.1932) centre (-48.3213, 19.6932) ccw
  arc A250 (-45.9, 18.7719) -> (-46.3393, 19.8325) centre (-47.4, 18.7719) ccw
  arc A251 (-47.2607, 58.7539) -> (-48.3213, 59.1932) centre (-48.3213, 57.6932) ccw
  arc A252 (-45.9, 56.7719) -> (-46.3393, 57.8325) centre (-47.4, 56.7719) ccw
  arc A253 (-42.5393, 62.3325) -> (-41.4787, 61.8932) centre (-41.4787, 63.3932) ccw
  arc A254 (-43.9, 64.3145) -> (-43.4607, 63.2539) centre (-42.4, 64.3145) ccw
  arc A255 (-122.3393, 56.2539) -> (-121.9, 57.3145) centre (-123.4, 57.3145) ccw
  arc A256 (-124.3213, 54.8932) -> (-123.2607, 55.3325) centre (-124.3213, 56.3932) ccw
  arc A257 (-117.4787, 52.1932) -> (-118.5393, 51.7539) centre (-117.4787, 50.6932) ccw
  arc A258 (-119.4607, 50.8325) -> (-119.9, 49.7719) centre (-118.4, 49.7719) ccw
  arc A259 (-122.3393, 37.2539) -> (-121.9, 38.3145) centre (-123.4, 38.3145) ccw
  arc A260 (-124.3213, 35.8932) -> (-123.2607, 36.3325) centre (-124.3213, 37.3932) ccw
  arc A261 (-119.4607, 31.8325) -> (-119.9, 30.7719) centre (-118.4, 30.7719) ccw
  arc A262 (-117.4787, 33.1932) -> (-118.5393, 32.7539) centre (-117.4787, 31.6932) ccw
  dimension "d1" = 3.2
  dimension "d2" = 3.2
  dimension "d3" = 7
  dimension "d4" = 3.2
  dimension "d5" = 3.2
  dimension "d9" = 2.2
  dimension "d12" = 2.2
  constraint tangent L19 A5
  constraint tangent L19 A6
  constraint tangent L13 A7
  constraint tangent L17 A8
  constraint tangent L12 A9
  constraint tangent L16 A10
  constraint tangent L8 A11
  constraint tangent L7 A13
  constraint tangent L9 A14
  constraint tangent L18 A15
  constraint tangent L2 A16
  constraint tangent L0 A17
  constraint tangent L10 A18
  constraint tangent L5 A19
  constraint tangent L11 A20
  constraint tangent L6 A21
  constraint tangent L3 A22
  constraint tangent L1 A23
  constraint tangent L4 A24
  constraint tangent L15 A25
  constraint tangent A24 L104
  constraint perpendicular L104 L105
  constraint tangent L104 A26
  constraint tangent L105 A26
  constraint coincident L15.end L105
  constraint perpendicular L15 L105
  constraint coincident L14.end L104
  constraint perpendicular L14 L104
  constraint tangent L32 A27
  constraint tangent L33 A28
  constraint tangent L35 A29
  constraint tangent L34 A30
  constraint tangent L49 A31
  constraint tangent L49 A32
  constraint tangent L51 A33
  constraint tangent L50 A34
  constraint tangent L57 A35
  constraint tangent L57 A36
  constraint tangent L59 A37
  constraint tangent L58 A38
  constraint tangent L76 A39
  constraint tangent L78 A40
  constraint tangent L79 A41
  constraint tangent L77 A42
  constraint tangent L54 A43
  constraint tangent L54 A44
  constraint tangent L52 A45
  constraint tangent L53 A46
  constraint tangent L90 A47
  constraint tangent L90 A48
  constraint tangent L91 A48
  constraint tangent L91 A49
  constraint tangent L89 A50
  constraint tangent L100 A51
  constraint tangent L101 A52
  constraint tangent L103 A53
  constraint tangent L102 A54
  constraint tangent L93 A55
  constraint tangent L93 A56
  constraint tangent L95 A57
  constraint tangent L94 A58
  constraint tangent L21 A59
  constraint tangent L20 A60
  constraint tangent L22 A60
  constraint tangent L22 A61
  constraint tangent L23 A62
  constraint tangent L64 A63
  constraint tangent L66 A63
  constraint tangent L64 A64
  constraint tangent L65 A65
  constraint tangent L67 A66
  constraint tangent L98 A67
  constraint tangent L98 A68
  constraint tangent L96 A69
  constraint tangent L97 A70
  constraint tangent L70 A71
  constraint tangent L70 A72
  constraint tangent L68 A73
  constraint tangent L69 A74
  constraint tangent L80 A75
  constraint tangent L80 A76
  constraint tangent L82 A76
  constraint tangent L82 A77
  constraint tangent L83 A77
  constraint tangent L83 A78
  constraint tangent L81 A78
  constraint tangent L29 A79
  constraint tangent L29 A80
  constraint tangent L28 A81
  constraint tangent L30 A82
  constraint tangent L37 A83
  constraint tangent L37 A84
  constraint tangent L36 A84
  constraint tangent L36 A85
  constraint tangent L38 A85
  constraint tangent L38 A86
  constraint tangent L39 A86
  constraint tangent L61 A87
  constraint tangent L61 A88
  constraint tangent L60 A88
  constraint tangent L60 A89
  constraint tangent L62 A90
  constraint tangent L40 A91
  constraint tangent L42 A92
  constraint tangent L43 A93
  constraint tangent L41 A93
  constraint tangent L41 A94
  constraint tangent L40 A94
  constraint tangent L44 A95
  constraint tangent L46 A95
  constraint tangent L46 A96
  constraint tangent L47 A96
  constraint tangent L47 A97
  constraint tangent L45 A97
  constraint tangent L45 A98
  constraint tangent L44 A98
  constraint tangent L74 A99
  constraint tangent L75 A99
  constraint tangent L74 A100
  constraint tangent L72 A101
  constraint tangent L73 A102
  constraint tangent L26 A103
  constraint tangent L27 A103
  constraint tangent L26 A104
  constraint tangent L24 A105
  constraint tangent L25 A106
  constraint tangent L86 A107
  constraint tangent L87 A107
  constraint tangent L86 A108
  constraint tangent L84 A109
  constraint tangent L85 A110
  constraint concentric A26 A132
  constraint concentric A24 A133
  constraint concentric A15 A134
  constraint concentric A14 A135
  constraint tangent A134 L130
  constraint tangent A132 L127
  constraint tangent L127 A133
  constraint tangent L129 A134
  constraint tangent L130 A135
  constraint coincident L114 L131.start
  constraint coincident L127 L131.end
  constraint perpendicular L127 L131
  constraint coincident L113 L132.start
  constraint perpendicular L113 L133
  constraint coincident L113 L133.end
  constraint perpendicular L133 L134
  constraint coincident L114 L135.end
  constraint tangent L136 A138
  constraint tangent L134 A138
  constraint tangent L133 A139
  constraint tangent L134 A139
  constraint tangent L135 A140
  constraint tangent L136 A140
  constraint coincident L114 L137.start
  constraint perpendicular L104 L137
  constraint perpendicular L137 L138
  constraint perpendicular L114 L139
  constraint coincident L114 L139.end
  constraint tangent L137 A141
  constraint tangent L138 A141
  constraint tangent L138 A142
  constraint tangent L139 A142
  constraint concentric A12 A111
  constraint concentric A11 A112
  constraint concentric A10 A113
  constraint concentric A9 A114
  constraint concentric A8 A115
  constraint concentric A7 A116
  constraint concentric A6 A117
  constraint concentric A5 A118
  constraint concentric A26 A119
  constraint concentric A24 A120
  constraint concentric A23 A121
  constraint concentric A22 A122
  constraint concentric A21 A123
  constraint concentric A20 A124
  constraint concentric A19 A125
  constraint concentric A18 A126
  constraint concentric A17 A127
  constraint concentric A16 A128
  constraint concentric A15 A129
  constraint concentric A14 A130
  constraint concentric A13 A131
  constraint tangent L124 A130
  constraint tangent L106 A131
  constraint tangent L123 A129
  constraint tangent A112 L107
  constraint tangent A113 L108
  constraint tangent A117 L112
  constraint tangent A129 L124
  constraint tangent A114 L109
  constraint tangent A115 L110
  constraint tangent A116 L111
  constraint tangent L112 A118
  constraint tangent A120 L115
  constraint tangent L113 A119
  constraint tangent A119 L114
  constraint tangent L114 A120
  constraint tangent A121 L116
  constraint tangent A122 L117
  constraint tangent A126 L121
  constraint tangent A123 L118
  constraint tangent A124 L119
  constraint tangent A125 L120
  constraint tangent A127 L122
  constraint tangent A128 L123
  constraint tangent A130 L125
  constraint tangent A12 L141
  constraint parallel L140 L142
  constraint tangent A111 L143
  constraint tangent L143 A143
  constraint tangent L142 A143
  constraint tangent L140 A144
  constraint tangent L141 A144
  constraint horizontal L144
  constraint tangent L144 A145
  constraint tangent L144 A146
  constraint tangent A135 L146
  constraint tangent A132 L149
  constraint horizontal L150
  constraint horizontal L151
  constraint concentric A8 A147
  constraint concentric A6 A148
  constraint concentric A23 A149
  constraint concentric A21 A150
  constraint parallel L152 L245
  constraint tangent A151 L245
  constraint tangent L153 A151
  constraint tangent L152 A152
  constraint tangent L152 A153
  constraint tangent L153 A153
  constraint parallel L154 L253
  constraint tangent A156 L253
  constraint tangent L155 A156
  constraint tangent A154 L154
  constraint tangent L154 A155
  constraint tangent A155 L155
  constraint horizontal L156
  constraint perpendicular L156 L157
  constraint parallel L156 L158
  constraint parallel L157 L159
  constraint tangent A160 L159
  constraint tangent L158 A160
  constraint tangent A157 L156
  constraint tangent A157 L159
  constraint tangent L156 A158
  constraint tangent A158 L157
  constraint tangent L157 A159
  constraint tangent A159 L158
  constraint horizontal L160
  constraint perpendicular L160 L161
  constraint parallel L160 L162
  constraint parallel L161 L163
  constraint tangent A164 L163
  constraint tangent L162 A164
  constraint tangent A161 L160
  constraint tangent A161 L163
  constraint tangent L160 A162
  constraint tangent A162 L161
  constraint tangent L161 A163
  constraint tangent A163 L162
  constraint horizontal L164
  constraint perpendicular L164 L248
  constraint parallel L165 L248
  constraint tangent A167 L165
  constraint tangent A165 L164
  constraint tangent A165 L165
  constraint tangent L164 A166
  constraint tangent A166 L248
  constraint horizontal L166
  constraint perpendicular L166 L251
  constraint parallel L167 L251
  constraint tangent A170 L167
  constraint tangent A168 L166
  constraint tangent A168 L167
  constraint tangent L166 A169
  constraint tangent A169 L251
  constraint horizontal L168
  constraint perpendicular L168 L169
  constraint parallel L168 L170
  constraint parallel L169 L171
  constraint tangent A174 L171
  constraint tangent L170 A174
  constraint tangent A171 L168
  constraint tangent A171 L171
  constraint tangent L168 A172
  constraint tangent A172 L169
  constraint tangent L169 A173
  constraint tangent A173 L170
  constraint horizontal L172
  constraint perpendicular L172 L173
  constraint parallel L172 L174
  constraint parallel L173 L175
  constraint tangent A178 L175
  constraint tangent L174 A178
  constraint tangent A175 L172
  constraint tangent A175 L175
  constraint tangent L172 A176
  constraint tangent A176 L173
  constraint tangent L173 A177
  constraint tangent A177 L174
  constraint horizontal L176
  constraint perpendicular L176 L177
  constraint parallel L176 L178
  constraint parallel L177 L179
  constraint tangent A182 L179
  constraint tangent L178 A182
  constraint tangent A179 L176
  constraint tangent A179 L179
  constraint tangent L176 A180
  constraint tangent A180 L177
  constraint tangent L177 A181
  constraint tangent A181 L178
  constraint horizontal L188
  constraint perpendicular L188 L189
  constraint parallel L188 L190
  constraint parallel L189 L191
  constraint tangent A194 L191
  constraint tangent L190 A194
  constraint tangent A191 L188
  constraint tangent A191 L191
  constraint tangent L188 A192
  constraint tangent A192 L189
  constraint tangent L189 A193
  constraint tangent A193 L190
  constraint horizontal L184
  constraint perpendicular L184 L185
  constraint parallel L184 L186
  constraint parallel L185 L187
  constraint tangent A190 L187
  constraint tangent L186 A190
  constraint tangent A187 L184
  constraint tangent A187 L187
  constraint tangent L184 A188
  constraint tangent A188 L185
  constraint tangent L185 A189
  constraint tangent A189 L186
  constraint horizontal L180
  constraint perpendicular L180 L181
  constraint parallel L180 L182
  constraint parallel L181 L183
  constraint tangent A186 L183
  constraint tangent L182 A186
  constraint tangent A183 L180
  constraint tangent A183 L183
  constraint tangent L180 A184
  constraint tangent A184 L181
  constraint tangent L181 A185
  constraint tangent A185 L182
  constraint horizontal L198
  constraint perpendicular L198 L199
  constraint parallel L198 L200
  constraint parallel L199 L201
  constraint tangent A205 L201
  constraint tangent L200 A205
  constraint tangent A202 L198
  constraint tangent A202 L201
  constraint tangent L198 A203
  constraint tangent A203 L199
  constraint tangent L199 A204
  constraint tangent A204 L200
  constraint horizontal L196
  constraint perpendicular L196 L197
  constraint parallel L196 L240
  constraint tangent A199 L196
  constraint tangent L196 A200
  constraint tangent A200 L197
  constraint tangent L197 A201
  constraint tangent A201 L240
  constraint horizontal L192
  constraint perpendicular L192 L193
  constraint parallel L192 L194
  constraint parallel L193 L195
  constraint tangent A198 L195
  constraint tangent L194 A198
  constraint tangent A195 L192
  constraint tangent A195 L195
  constraint tangent L192 A196
  constraint tangent A196 L193
  constraint tangent L193 A197
  constraint tangent A197 L194
  constraint horizontal L202
  constraint perpendicular L202 L203
  constraint parallel L202 L237
  constraint tangent A206 L202
  constraint tangent L202 A207
  constraint tangent A207 L203
  constraint tangent L203 A208
  constraint tangent A208 L237
  constraint horizontal L242
  constraint perpendicular L214 L242
  constraint parallel L215 L242
  constraint parallel L214 L216
  constraint tangent A222 L216
  constraint tangent L215 A222
  constraint tangent A220 L242
  constraint tangent A220 L216
  constraint tangent L214 A221
  constraint tangent A221 L215
  constraint horizontal L210
  constraint perpendicular L210 L211
  constraint parallel L210 L212
  constraint parallel L211 L213
  constraint tangent A219 L213
  constraint tangent L212 A219
  constraint tangent A216 L210
  constraint tangent A216 L213
  constraint tangent L210 A217
  constraint tangent A217 L211
  constraint tangent L211 A218
  constraint tangent A218 L212
  constraint horizontal L235
  constraint parallel L208 L235
  constraint tangent A215 L209
  constraint tangent L208 A215
  constraint tangent A213 L235
  constraint tangent A213 L209
  constraint tangent A214 L208
  constraint horizontal L204
  constraint perpendicular L204 L205
  constraint parallel L204 L206
  constraint parallel L205 L207
  constraint tangent A212 L207
  constraint tangent L206 A212
  constraint tangent A209 L204
  constraint tangent A209 L207
  constraint tangent L204 A210
  constraint tangent A210 L205
  constraint tangent L205 A211
  constraint tangent A211 L206